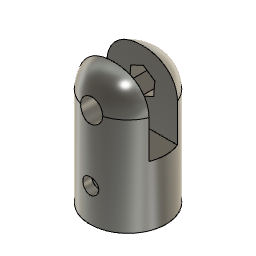
_Selfy Stick head.3965dfcc-8473-4542-a756-688ec4b2d722_LV2 (Autodesk Fusion 360 design; units mm, degrees)
Autodesk Fusion 360 part; units mm, degrees
sketch "Sketch1" plane through (0, 0, 0) normal (0, 0, 1) x (1, 0, 0) in component "Base"
  circle A0 centre (0, 0) radius 12
  dimension "d33" = 24
  constraint coincident A0.centre origin
  measures "d33" diameter of A0
extrude "Extrude1" add sketch "Sketch1" along normal blind 41 in component "Base"
ref_plane "WorkPlane1" through (0, -12, 17.2236) normal (0, -1, 0) x (-1, 0, 0) in component "Base"
sketch "Sketch2" plane through (0, -12, 17.2236) normal (0, -1, 0) x (1, 0, 0) in component "Base"
  line L0 (12, -17.2236) -> (-12, -17.2236)
  line L1 (12, 23.7764) -> (-12, 23.7764)
  line L2 (-17.778, -9.2236) -> (25, -9.2236) construction
  line L3 (-17.5615, 10.2764) -> (25, 10.2764) construction
  circle A0 centre (-0.0008, -6.7236) radius 2.5
  circle A1 centre (-0.0008, -6.7236) radius 1.5
  circle A2 centre (-0.0002, 13.7764) radius 3.5
  dimension "d37" = 24
  dimension "d38" = 41
  dimension "d39" = 8
  dimension "d40" = 27.5
  dimension "d42" = 5
  dimension "d43" = 10.5
  dimension "d44" = 3
  dimension "d45" = 7
  dimension "d46" = 31
  constraint horizontal L2
  constraint horizontal L3
  constraint concentric A0 A1
  measures "d37" distance of L0.start L0.end
  measures "d38" distance of L0 L1
  measures "d39" distance of L0 L2
  measures "d40" distance of L0 L3
  measures "d42" diameter of A0
  measures "d43" distance of L0 A0.centre
  measures "d44" diameter of A1
  measures "d45" diameter of A2
  measures "d46" distance of L0 A2.centre
extrude "Extrude2" cut sketch "Sketch2" against normal blind 24 contours A1 | A2 in component "Base"
ref_plane "WorkPlane2" through (0, -12, 12.6145) normal (0, -1, 0) x (-1, 0, 0) in component "Base"
sketch "Sketch3" plane through (0, -12, 12.6145) normal (0, -1, 0) x (1, 0, 0) in component "Base"
  line L0 (12, -12.6145) -> (-12, -12.6145)
  circle A0 centre (0, -2.1) radius 2.5
  dimension "d51" = 5
  measures "d51" diameter of A0
extrude "Extrude3" cut sketch "Sketch3" against normal blind 3 in component "Base"
fillet "Fillet1" radius 10 1 edges at (-11.1879, -4.3394, 41) in component "Base"
ref_plane "WorkPlane6" through (0, 0, 41) normal (0, 0, 1) x (1, 0, 0) in component "Base"
sketch "Sketch4" plane through (0, 0, 41) normal (0, 0, 1) x (1, 0, 0) in component "Base"
  line L0 (-14, 4.5) -> (14, 4.5)
  line L1 (14, 4.5) -> (14, -4.5)
  line L2 (14, -4.5) -> (-14, -4.5)
  line L3 (-14, -4.5) -> (-14, 4.5)
  line L4 (-14, 4.5) -> (14, -4.5) construction
  line L5 (14, 4.5) -> (-14, -4.5) construction
  dimension "d60" = 9
  constraint horizontal L0
  constraint perpendicular L0 L1
  constraint parallel L0 L2
  constraint parallel L1 L3
  constraint coincident L4 origin
  constraint coincident L5 origin
  measures "d60" distance of L0.end L1.end
extrude "Extrude4" cut sketch "Sketch4" against normal blind 22 in component "Base"
ref_plane "WorkPlane7" through (0, 12, 20.5561) normal (0, 1, 0) x (1, 0, 0) in component "Base"
sketch "Sketch5" plane through (0, 12, 20.5561) normal (0, 1, 0) x (1, 0, 0) in component "Base"
  line L0 (-3.628, -12.9566) -> (0.3454, -14.8465)
  line L1 (0.3454, -14.8465) -> (3.9689, -12.3504)
  line L2 (3.9689, -12.3504) -> (3.6189, -7.9643)
  line L3 (3.6189, -7.9643) -> (-0.3546, -6.0744)
  line L4 (-0.3546, -6.0744) -> (-3.978, -8.5706)
  line L5 (-3.978, -8.5706) -> (-3.628, -12.9566)
  point P0 (-0.0046, -10.4605)
  dimension "d64" = 4.4
  measures "d64" distance of L0.start P0
extrude "Extrude5" cut sketch "Sketch5" against normal up to surface (7.5 mm away) in component "Base"
ref_plane "WorkPlane8" through (0, 12, 4.5743) normal (0, 1, 0) x (1, 0, 0) in component "Base"
sketch "Sketch6" plane through (0, 12, 4.5743) normal (0, 1, 0) x (1, 0, 0) in component "Base"
  circle A0 centre (-0.0008, -5.9257) radius 1.5
  line L0 (-2.8139, -4.6232) -> (-2.5353, -7.7106)
  line L1 (-2.5353, -7.7106) -> (0.2778, -9.0131)
  line L2 (0.2778, -9.0131) -> (2.8123, -7.2282)
  line L3 (2.8123, -7.2282) -> (2.5338, -4.1407)
  line L4 (2.5338, -4.1407) -> (-0.2793, -2.8382)
  line L5 (-0.2793, -2.8382) -> (-2.8139, -4.6232)
  point P0 (-0.0008, -5.9257)
  dimension "d68" = 3
  dimension "d69" = 3.1
  constraint coincident P0 A0.centre
  measures "d68" diameter of A0
  measures "d69" distance of L0.start P0
extrude "Extrude6" cut sketch "Sketch6" against normal blind 2.6 in component "Base"
ref_plane "WorkPlane10" through (0, 0, 0) normal (0, 0, -1) x (-1, 0, 0) in component "Base"
sketch "Sketch7" plane through (0, 0, 0) normal (0, 0, -1) x (1, 0, 0) in component "Base"
  circle A0 centre (0, 0) radius 6.5
  dimension "d74" = 13
  constraint coincident A0.centre origin
  measures "d74" diameter of A0
extrude "Extrude7" cut sketch "Sketch7" against normal blind 18 in component "Base"
component "Top bottom half" placed x (1, 0, 0) y (0, 1, 0) z (0, 0, 1) at (0, 0, 0)
component "Base" placed x (1, 0, 0) y (0, 1, 0) z (0, 0, 1) at (0, 0, 0)
